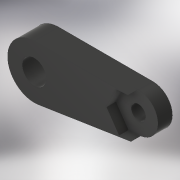
# Autodesk Inventor part: TA07
Saved by Autodesk Inventor 2017 (Build 210142000, 142)
## iProperties
Created: 2019-04-10
Part Number: TA07
Material: ABS Plastic
Document SubType Name: Modeling
Designer: Dell
Density: 1.06 g/cm^3
Appearance: Smooth - Black
Author: Dell
Autodesk Inventor part; units mm, degrees
ref_plane "YZ Plane" through (0, 0, 0) normal (1, 0, 0) x (0, 1, 0)
ref_plane "XZ Plane" through (0, 0, 0) normal (0, 1, 0) x (-1, 0, 0)
ref_plane "XY Plane" through (0, 0, 0) normal (0, 0, 1) x (1, 0, 0)
sketch "Sketch1" plane through (0, 0, 0) normal (0, 0, 1) x (1, 0, 0)
  circle A0 centre (0, 0) radius 2.5
  circle A1 centre (0, 0) radius 5.5
  circle A2 centre (19.4422, 1.5) radius 1.5
  circle A3 centre (19.4422, 1.5) radius 4
  line L0 (0, 5.5) -> (19.4422, 5.5)
  line L1 (20.0558, -2.4527) -> (0.8436, -5.4349)
  point P0 (22.8922, -0.5243)
  dimension "d0" = 5
  dimension "d1" = 11
  dimension "d2" = 3
  dimension "d3" = 8
  dimension "d4" = 19.5
  constraints: 5 point on circle, 4 centre point, 4 end point, 4 tangent, 3 coincident, 1 horizontal
  measures "d0" diameter of A0
  measures "d1" diameter of A1
  measures "d2" diameter of A2
  measures "d3" diameter of A3
  measures "d4" distance of A2.centre point (0, 0)
extrude "Extrusion1" add sketch "Sketch1" along normal blind 5
sketch "Sketch2" plane through (0, 0, 5) normal (0, 0, 1) x (1, 0, 0)
  circle A0 centre (19.4422, 1.5) radius 1.5 projected
  line L0 (24.0473, 1.8553) -> (22.0525, -2.3105)
  line L1 (22.0525, -2.3105) -> (17.4474, -2.6658)
  line L2 (17.4474, -2.6658) -> (14.8371, 1.1447)
  line L3 (14.8371, 1.1447) -> (16.832, 5.3105)
  line L4 (16.832, 5.3105) -> (21.4371, 5.6658)
  line L5 (21.4371, 5.6658) -> (24.0473, 1.8553)
  line L6 (0, 0) -> (19.4422, 1.5)
  dimension "d7" = 8
  constraints: 14 end point, 2 coincident, 1 point on line, 13 other
  measures "d7" distance between parallel lines of L1 L4
extrude "Extrusion2" cut sketch "Sketch2" against normal blind 2
body "Solid1"
